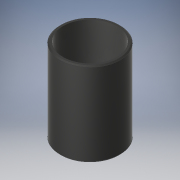
# Autodesk Inventor part: Part9
Saved by Autodesk Inventor 2019 (Build 230136000, 136)
## iProperties
Created: 2018-11-25
Part Number: Part9
Material: Acetal Resin, Black
Document SubType Name: Modeling
Designer: aleks
Density: 1.425 g/cm^3
Appearance: Smooth - Black
Author: aleks
Autodesk Inventor part; units mm, degrees
ref_plane "YZ Plane" through (0, 0, 0) normal (1, 0, 0) x (0, 1, 0)
ref_plane "XZ Plane" through (0, 0, 0) normal (0, 1, 0) x (-1, 0, 0)
ref_plane "XY Plane" through (0, 0, 0) normal (0, 0, 1) x (1, 0, 0)
sketch "Sketch1" plane through (0, 0, 0) normal (0, 1, 0) x (-1, 0, 0)
  circle A0 centre (0, 0) radius 5
  circle A1 centre (0, 0) radius 4.5
  dimension "d0" = 10
  dimension "d1" = 9
  constraints: 2 centre point, 2 coincident
  measures "d0" diameter of A0
  measures "d1" diameter of A1
extrude "Extrusion1" add sketch "Sketch1" along normal blind 14
chamfer "Chamfer1" distance 0.2 angle 45 1 edges at (5, 14, 0)
chamfer "Chamfer2" distance 0.2 angle 45 1 edges at (5, 0, 0)
body "Solid1"
